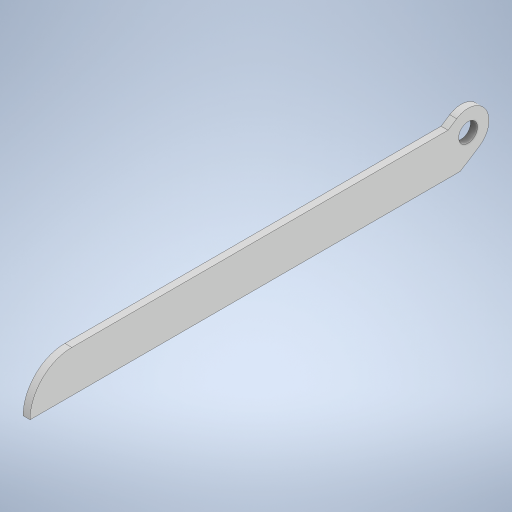
# Autodesk Inventor part: filo
Saved by Autodesk Inventor 2023 (Build 270158000, 158)
## iProperties
Created: 2022-04-05
Part Number: filo
Material: Genérico
Document SubType Name: Modeling
Designer: isaac
Density: 1 g/cm^3
Appearance: Valor por defecto
Author: isaac
Autodesk Inventor part; units mm, degrees
ref_plane "YZ Plane" through (0, 0, 0) normal (1, 0, 0) x (0, 1, 0)
ref_plane "XZ Plane" through (0, 0, 0) normal (0, 1, 0) x (-1, 0, 0)
ref_plane "XY Plane" through (0, 0, 0) normal (0, 0, 1) x (1, 0, 0)
sketch "Boceto1" plane through (0, 0, 0) normal (1, 0, 0) x (0, 1, 0)
  line L0 (0, 0) -> (0, 610)
  arc A0 (60, 550) -> (0, 610) centre (0, 550) ccw
  line L1 (60, 550) -> (60, 9.3292)
  line L2 (60, 9.3292) -> (68.06, -3.121)
  arc A1 (17.6931, -35.7275) -> (68.06, -3.121) centre (42.8766, -19.4242) ccw
  line L3 (17.6931, -35.7275) -> (0, -8.3971)
  line L4 (0, -8.3971) -> (0, 0)
  circle A2 centre (42.8766, -19.4242) radius 13.5
  dimension "d1" = 60
  dimension "d2" = 550
  dimension "d6" = 60
  dimension "d7" = 30
  dimension "d8" = 27
  dimension "d10" = 42.8766
  dimension "d11" = 19.4242
  dimension "d12" = 32.5576
  constraints: 10 end point, 4 point on circle, 3 centre point, 2 parallel, 2 tangent, 2 vertical, 1 coincident, 1 point on line
  measures "d1" distance between parallel lines of L0 L1
  measures "d2" distance of L0.start A0.centre
  measures "d6" radius of A0
  measures "d7" radius of A1
  measures "d8" diameter of A2
  measures "d10" horizontal distance of L0.start A1.centre
  measures "d11" vertical distance of L0.start A1.centre
  measures "d12" distance of L3.start L3.end
extrude "Extrusión1" add sketch "Boceto1" along normal blind 10
